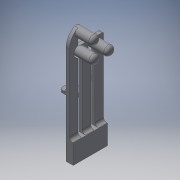
# Autodesk Inventor part: Level1_CPY
Saved by Autodesk Inventor 2016 (Build 200138000, 138)
## iProperties
Created: 2016-04-09
Part Number: Level1_CPY
Material: Generic
Document SubType Name: Modeling
Designer: Vijay
Density: 1 g/cm^3
Appearance: Default
Author: Vijay
Autodesk Inventor part; units mm, degrees
ref_plane "YZ Plane" through (0, 0, 0) normal (1, 0, 0) x (0, 1, 0)
ref_plane "XZ Plane" through (0, 0, 0) normal (0, 1, 0) x (-1, 0, 0)
ref_plane "XY Plane" through (0, 0, 0) normal (0, 0, 1) x (1, 0, 0)
sketch "Sketch1" plane through (0, 0, 0) normal (1, 0, 0) x (0, 1, 0)
  circle A0 centre (4.3679, -6.0703) radius 0.7 construction
  circle A1 centre (4.3679, -8.3603) radius 0.7 construction
  circle A2 centre (6.9079, -6.0703) radius 0.7 construction
  arc A3 (5.0679, -6.0703) -> (3.6834, -6.2166) centre (4.3679, -6.0703) ccw
  arc A4 (5.0679, -8.3603) -> (3.6772, -8.2466) centre (4.3679, -8.3603) ccw
  arc A5 (6.2089, -6.0338) -> (7.5634, -5.8248) centre (6.9079, -6.0703) ccw
  line L0 (14.3238, -4.4653) -> (-0.6762, -4.4653) construction
  line L1 (-0.6762, -9.9653) -> (14.3238, -9.9653) construction
  line L2 (-4.7504, -8.4142) -> (3.4798, -8.4142)
  line L3 (5.0679, -8.3603) -> (5.0679, -9.535)
  line L4 (4.8679, -9.735) -> (-4.7504, -9.735)
  line L5 (-4.7504, -9.735) -> (-4.7504, -8.4142)
  line L6 (-4.7504, -7.7792) -> (-4.7504, -6.4584)
  line L7 (-4.7504, -6.4584) -> (3.4878, -6.4584)
  line L8 (5.0679, -6.0703) -> (5.0679, -7.2585)
  line L9 (-4.7298, -5.8234) -> (-4.7298, -4.5026)
  line L10 (-4.7298, -4.5026) -> (5.4352, -4.5026)
  line L11 (7.5634, -5.8234) -> (7.5634, -5.8248)
  arc A6 (6.2089, -6.0338) -> (6.0091, -5.8234) centre (6.0091, -6.0234) ccw
  arc A7 (5.159, -5.7069) -> (3.5768, -5.7069) centre (4.3679, -6.0703) ccw
  line L12 (6.0091, -5.8234) -> (5.3407, -5.8234)
  line L13 (3.3951, -5.8234) -> (-4.7298, -5.8234)
  arc A8 (5.159, -5.7069) -> (5.3407, -5.8234) centre (5.3407, -5.6234) ccw
  arc A9 (3.3951, -5.8234) -> (3.5768, -5.7069) centre (3.3951, -5.6234) ccw
  arc A10 (3.4878, -6.4584) -> (3.6834, -6.2166) centre (3.4878, -6.2584) ccw
  arc A11 (3.4798, -8.4142) -> (3.6772, -8.2466) centre (3.4798, -8.2142) ccw
  arc A12 (5.0621, -7.6269) -> (5.0679, -7.5792) centre (4.8679, -7.5792) ccw
  arc A13 (4.8679, -9.735) -> (5.0679, -9.535) centre (4.8679, -9.535) ccw
  arc A14 (4.7852, -7.4407) -> (3.5967, -7.7083) centre (4.3679, -8.3603) ccw
  line L14 (3.4439, -7.7792) -> (-4.7504, -7.7792)
  arc A15 (4.7852, -7.4407) -> (5.0679, -7.2585) centre (4.8679, -7.2585) ccw
  arc A16 (3.4439, -7.7792) -> (3.5967, -7.7083) centre (3.4439, -7.5792) ccw
  arc A17 (7.5634, -5.8248) -> (5.2328, -4.5026) centre (5.334, -7.0394) ccw
  point P0 (6.2524, -5.8248)
  point P1 (5.2027, -5.8234)
  point P2 (3.5331, -5.8234)
  point P3 (3.7853, -6.4584)
  point P4 (3.67, -8.4142)
  point P5 (3.542, -7.7792)
  dimension "d9" = 0.2
  dimension "d10" = 0.2
  dimension "d11" = 0.2
  dimension "d12" = 1.3208
  dimension "d13" = 1.3208
  dimension "d14" = 1.3208
  dimension "d15" = 0.2
  dimension "d16" = 0.635
  dimension "d17" = 0.635
  constraints: 40 point on circle, 26 end point, 19 tangent, 15 centre point, 8 point on line, 7 parallel, 5 coincident, 5 equal radius, 4 horizontal, 4 perpendicular, 4 other
  measures "d9" radius of A6
  measures "d10" radius of A8
  measures "d11" radius of A10
  measures "d12" distance of L9.start L9.end
  measures "d13" distance of L6.start L6.end
  measures "d14" distance of L4.end L2.start
  measures "d15" radius of A15
  measures "d16" distance between parallel lines of L7 L13
  measures "d17" distance between parallel lines of L2 L14
extrude "Extrusion1" add sketch "Sketch1" along normal blind 0.5
sketch "Sketch2" plane through (0.5, 0, 0) normal (1, 0, 0) x (0, 0, -1)
  arc A0 (6.0338, 6.2089) -> (5.8248, 7.5634) centre (6.0703, 6.9079) ccw construction
  arc A1 (6.0703, 5.0679) -> (6.2166, 3.6834) centre (6.0703, 4.3679) ccw construction
  arc A2 (8.3603, 5.0679) -> (8.2466, 3.6772) centre (8.3603, 4.3679) ccw construction
  circle A3 centre (6.0703, 4.3679) radius 0.7
  circle A4 centre (6.0703, 6.9079) radius 0.7
  circle A5 centre (8.3603, 4.3679) radius 0.7
  point P0 (0, 0)
  constraints: 3 centre point, 3 coincident, 2 concentric
ref_plane "Work Plane1" through (3.5, -15.6321, -16.2153) normal (1, 0, 0) x (0, 1, 0)
ref_plane "Work Plane2" through (3.1, -15.6321, -16.2153) normal (1, 0, 0) x (0, 1, 0)
extrude "Extrusion2" add sketch "Sketch2" along normal up to surface (2.6 mm away)
fillet "Fillet1" radius 0.5 3 edges at (3.1, 4.3679, -5.3703) (3.1, 4.3679, -7.6603) (3.1, 6.9079, -5.3703)
sketch "Sketch3" plane through (0, -4.7298, -5.8234) normal (0, -1, 0) x (1, 0, 0)
  line L0 (0, 1.3208) -> (0, 0) projected
  line L1 (0, 0) -> (0.5, 0) projected
  line L2 (0.5, 1.3208) -> (0.5, 0) projected
  line L3 (0, 1.3208) -> (0.5, 1.3208) projected
  line L4 (0, -0.635) -> (0, -1.9558) projected
  line L5 (0, -1.9558) -> (0.5, -1.9558) projected
  line L6 (0.5, -0.635) -> (0.5, -1.9558) projected
  line L7 (0, -0.635) -> (0.5, -0.635) projected
  line L8 (0, -3.9116) -> (0, -2.5908) projected
  line L9 (0, -3.9116) -> (0.5, -3.9116) projected
  line L10 (0.5, -2.5908) -> (0.5, -3.9116) projected
  line L11 (0, -2.5908) -> (0.5, -2.5908) projected
  point P0 (0, 5.8234)
extrude "Extrusion3" add sketch "Sketch3" along normal blind 5
sketch "Sketch4" plane through (0, 0, 0) normal (-1, 0, 0) x (0, 0, 1)
  arc A0 (-4.5026, 5.4352) -> (-5.8248, 7.5634) centre (-7.0394, 5.334) ccw projected
  arc A1 (-5.8248, 7.5634) -> (-6.0338, 6.2089) centre (-6.0703, 6.9079) ccw projected
  arc A2 (-5.8234, 6.0091) -> (-6.0338, 6.2089) centre (-6.0234, 6.0091) ccw projected
  line L0 (-5.8234, 5.3407) -> (-5.8234, 6.0091) projected
  arc A3 (-5.8234, 5.3407) -> (-5.7069, 5.159) centre (-5.6234, 5.3407) ccw projected
  arc A4 (-5.7069, 3.5768) -> (-5.7069, 5.159) centre (-6.0703, 4.3679) ccw projected
  arc A5 (-5.7069, 3.5768) -> (-5.8234, 3.3951) centre (-5.6234, 3.3951) ccw projected
  line L1 (-5.8234, 3.3951) -> (-5.8234, -9.7298) projected
  line L2 (-4.5026, -9.7298) -> (-5.8234, -9.7298) projected
  line L3 (-4.5026, 5.4352) -> (-4.5026, -9.7298) projected
  line L4 (-6.4584, 3.4878) -> (-6.4584, -9.7298) projected
  arc A6 (-6.2166, 3.6834) -> (-6.4584, 3.4878) centre (-6.2584, 3.4878) ccw projected
  arc A7 (-6.2166, 3.6834) -> (-6.0703, 5.0679) centre (-6.0703, 4.3679) ccw projected
  line L5 (-7.2585, 5.0679) -> (-6.0703, 5.0679) projected
  arc A8 (-7.2585, 5.0679) -> (-7.4407, 4.7852) centre (-7.2585, 4.8679) ccw projected
  arc A9 (-7.7083, 3.5967) -> (-7.4407, 4.7852) centre (-8.3603, 4.3679) ccw projected
  arc A10 (-7.7083, 3.5967) -> (-7.7792, 3.4439) centre (-7.5792, 3.4439) ccw projected
  line L6 (-7.7792, 3.4439) -> (-7.7792, -9.7298) projected
  line L7 (-6.4584, -9.7298) -> (-7.7792, -9.7298) projected
  line L8 (-8.4142, -9.7298) -> (-8.4142, 3.4798) projected
  arc A11 (-8.2466, 3.6772) -> (-8.4142, 3.4798) centre (-8.2142, 3.4798) ccw projected
  arc A12 (-8.2466, 3.6772) -> (-8.3603, 5.0679) centre (-8.3603, 4.3679) ccw projected
  line L9 (-8.3603, 5.0679) -> (-9.535, 5.0679) projected
  arc A13 (-9.535, 5.0679) -> (-9.735, 4.8679) centre (-9.535, 4.8679) ccw projected
  line L10 (-9.735, 4.8679) -> (-9.735, -9.7298) projected
  line L11 (-8.4142, -9.7298) -> (-9.735, -9.7298) projected
  line L12 (-9.735, 4.8679) -> (-9.735, -9.7298) projected
  line L13 (-4.5026, -9.7298) -> (-9.735, -9.7298)
  line L14 (-9.735, -9.7298) -> (-9.735, -6.7298)
  line L15 (-9.735, -6.7298) -> (-4.5026, -6.7298)
  line L16 (-4.5026, -6.7298) -> (-4.5026, -9.7298)
  point P0 (0, 0)
  dimension "d25" = 3
  constraints: 8 end point, 2 parallel, 2 perpendicular
  measures "d25" distance between parallel lines of L13 L15
ref_plane "Work Plane3" through (1.1, -15.6321, -16.2153) normal (-1, 0, 0) x (0, 0, 1)
extrude "Extrusion4" add sketch "Sketch4" against normal up to surface (1.1 mm away) contours L3 L2 L1 L15 | L1 L13 L4 L15 | L4 L7 L6 L15 | L6 L13 L8 L15 | L8 L11 L10 L15
fillet "Fillet2" radius 0.5 3 edges at (0.5, -6.7298, -9.0746) (0.5, -6.7298, -7.1188) (0.5, -6.7298, -5.163)
sketch "Sketch5" plane through (0, 0, 0) normal (-1, 0, 0) x (0, 0, 1)
  line L0 (-5.2442, -1.1967) -> (-4.787, -0.2971) construction
  line L1 (-4.787, -0.2971) -> (-4.5061, -0.8188) construction
  arc A0 (-4.6135, -1.1015) -> (-4.5061, -0.8188) centre (-4.6822, -0.9136) ccw construction
  arc A1 (-5.2442, -1.1967) -> (-4.6135, -1.1015) centre (-5.163, 0.4012) ccw construction
  line L2 (-9.1666, -1.1961) -> (-8.7033, -0.2996) construction
  line L3 (-8.7033, -0.2996) -> (-8.4259, -0.8232) construction
  arc A2 (-8.5352, -1.1051) -> (-8.4259, -0.8232) centre (-8.6026, -0.9168) ccw construction
  arc A3 (-9.1666, -1.1961) -> (-8.5352, -1.1051) centre (-9.0746, 0.4012) ccw construction
  line L4 (-6.6258, -1.523) -> (-7.3007, -2.2732) construction
  line L5 (-7.3007, -2.2732) -> (-7.4367, -1.6965) construction
  arc A4 (-7.2596, -1.4514) -> (-7.4367, -1.6965) centre (-7.242, -1.6506) ccw construction
  arc A5 (-6.6258, -1.523) -> (-7.2596, -1.4514) centre (-7.1188, -3.0452) ccw construction
  line L6 (-9.735, 4.8679) -> (-9.735, -9.7298) projected
  line L7 (-9.735, -0.5988) -> (-8.4142, -0.5988)
  line L8 (-8.4142, -0.5988) -> (-8.4142, -0.9456)
  line L9 (-9.735, -0.9456) -> (-9.735, -0.5988)
  line L10 (-5.8234, -0.5988) -> (-4.5026, -0.5988)
  line L11 (-4.5026, -0.5988) -> (-4.5026, -0.9456)
  line L12 (-5.8234, -0.9456) -> (-5.8234, -0.5988)
  line L13 (-6.4584, -2.0452) -> (-7.7792, -2.0452)
  line L14 (-7.7792, -2.0452) -> (-7.7792, -1.6984)
  line L15 (-6.4584, -1.6984) -> (-6.4584, -2.0452)
  arc A6 (-9.735, -0.9456) -> (-8.4142, -0.9456) centre (-9.0746, 0.4012) ccw
  arc A7 (-5.8234, -0.9456) -> (-4.5026, -0.9456) centre (-5.163, 0.4012) ccw
  line L16 (-4.5026, 5.4352) -> (-4.5026, -9.7298) projected
  arc A8 (-6.4584, -1.6984) -> (-7.7792, -1.6984) centre (-7.1188, -3.0452) ccw
  point P0 (0, 0)
  dimension "d29" = 1
  dimension "d30" = 1
  constraints: 19 end point, 7 point on circle, 3 centre point, 3 coincident, 3 horizontal, 3 parallel, 3 perpendicular, 3 point on line, 1 collinear
  measures "d29" distance from line of A8.centre L13
  measures "d30" distance from line of L7 A3.centre
extrude "Extrusion5" add sketch "Sketch5" along normal blind 1
fillet "Fillet3" radius 0.4 6 edges at (-1, -0.7722, -8.4142) (-1, -0.7722, -9.735) (-1, -1.8718, -7.7792) (-1, -1.8718, -6.4584) (-1, -0.7722, -5.8234) (-1, -0.7722, -4.5026)
fillet "Fillet4" radius 0.4 3 edges at (0, -0.5988, -5.163) (0, -2.0452, -7.1188) (0, -0.5988, -9.0746)
body "Solid1"
